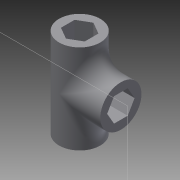
# Autodesk Inventor part: engancheBicsT
Saved by Autodesk Inventor 2015 SP1 (Build 190203100, 203)
## iProperties
Created: 2015-06-15
Part Number: engancheBicsT
Material: Genérico
Document SubType Name: Modeling
Designer: Javier
Density: 1 g/cm^3
Appearance: Valor por defecto
Author: Javier
Autodesk Inventor part; units mm, degrees
ref_plane "YZ Plane" through (0, 0, 0) normal (1, 0, 0) x (0, 1, 0)
ref_plane "XZ Plane" through (0, 0, 0) normal (0, 1, 0) x (-1, 0, 0)
ref_plane "XY Plane" through (0, 0, 0) normal (0, 0, 1) x (1, 0, 0)
sketch "Boceto1" plane through (0, 0, 0) normal (0, 0, 1) x (1, 0, 0)
  circle A0 centre (0, 0) radius 6
  line L0 (0, -4) -> (-3.4641, -2)
  line L1 (-3.4641, -2) -> (-3.4641, 2)
  line L2 (-3.4641, 2) -> (0, 4)
  line L3 (0, 4) -> (3.4641, 2)
  line L4 (3.4641, 2) -> (3.4641, -2)
  line L5 (3.4641, -2) -> (0, -4)
  dimension "d0" = 12
  dimension "d1" = 4
  constraints: 12 end point, 2 coincident, 1 centre point, 13 other
  measures "d0" diameter of A0
  measures "d1" distance of L3.end L4.end
extrude "Extrusión1" add sketch "Boceto1" along normal blind 7
sketch "Boceto2" plane through (0, 0, 7) normal (0, 0, 1) x (1, 0, 0)
  point P0 (0, 0)
sketch "Boceto3" plane through (0, 0, 7) normal (0, 0, 1) x (1, 0, 0)
  line L0 (-3.4641, -2) -> (-3.4641, 2) projected
  line L1 (-3.4641, 2) -> (0, 4) projected
  line L2 (0, 4) -> (3.4641, 2) projected
  line L3 (3.4641, 2) -> (3.4641, -2) projected
  line L4 (3.4641, -2) -> (0, -4) projected
  line L5 (0, -4) -> (-3.4641, -2) projected
  circle A0 centre (0, 0) radius 6 projected
extrude "Extrusión2" add sketch "Boceto3" along normal blind 12
ref_plane "Plano de trabajo1" through (0, -4, 19) normal (-1, 0, 0) x (0, 1, 0)
sketch "Boceto4" plane through (0, -4, 19) normal (-1, 0, 0) x (0, 1, 0)
  line L0 (8, 19) -> (8, 0) projected
  line L1 (0, 19) -> (0, 0) projected
  line L2 (6, 19) -> (2, 19) projected
  line L3 (6, 19) -> (6, 0) projected
  line L4 (2, 0) -> (6, 0) projected
  line L5 (2, 19) -> (2, 0) projected
  line L6 (2, 0) -> (6, 0)
  line L7 (4, 0) -> (4, 6)
  circle A0 centre (4, 6) radius 6
  line L8 (8, 6) -> (6, 2.5359)
  line L9 (6, 2.5359) -> (2, 2.5359)
  line L10 (2, 2.5359) -> (0, 6)
  line L11 (0, 6) -> (2, 9.4641)
  line L12 (2, 9.4641) -> (6, 9.4641)
  line L13 (6, 9.4641) -> (8, 6)
  circle A1 centre (4, 6) radius 4
  point P0 (4, 19)
  dimension "d6" = 6
  dimension "d7" = 12
  constraints: 16 end point, 3 coincident, 1 centre point, 1 midpoint, 1 perpendicular, 1 point on line, 1 vertical, 16 other
  measures "d6" distance of L7.start L7.end
  measures "d7" diameter of A0
extrude "Extrusión3" add sketch "Boceto4" against normal blind 12 contours A0 L0 | L0 A1 L3 A0 | L0 A0 L3 A1 | L3 A1 L5 A0 | L3 A0 L7 A1 | L5 A1 L1 A0 | L7 A0 L5 A1 | L1 A0 | L5 A0 L1 A1
sketch "Boceto7" plane through (0, 0, 19) normal (0, 0, 1) x (1, 0, 0)
  circle A0 centre (0, 0) radius 4
  point P0 (0, 4)
  constraints: 1 coincident, 1 vertical alignment, 2 other
extrude "Extrusión6" cut sketch "Boceto7" against normal blind 12
sketch "Boceto8" plane through (0, -4, 19) normal (-1, 0, 0) x (0, 1, 0)
  point P0 (4, 19)
sketch "Boceto9" plane through (12, 0, 13) normal (1, 0, 0) x (0, 0, -1)
  spline S0 degree 5 poles (-4, 0) (-3.9998, 1.0287) (-3.67, 2.0581) (-3.006, 2.9436) (-1.3134, 4.0903) (0.7107, 4.1022) (1.6429, 3.8257) (3.423, 2.6512) (4.2083, 0.6219) (4.2089, -0.6181) (3.4253, -2.6483) (1.6458, -3.8245) (0.7135, -4.1019) (-1.3114, -4.0911) (-3.0051, -2.9448) (-3.6697, -2.0589) (-3.9998, -1.0291) (-4, 0) knots 0 0 0 0 0 0 0.204671 0.204671 0.204671 0.387185 0.387185 0.387185 0.61267 0.61267 0.61267 0.795245 0.795245 0.795245 1 1 1 1 1 1 projected
  point P0 (13, 0)
  constraints: 1 other
extrude "Extrusión7" cut sketch "Boceto9" against normal blind 12
sketch "Boceto10" plane through (0, 0, 19) normal (0, 0, 1) x (1, 0, 0)
  circle A0 centre (0, 0) radius 6 projected
  line L0 (0, 4) -> (-3.4641, 2) projected
  line L1 (-3.4641, 2) -> (-3.4641, -2) projected
  line L2 (-3.4641, -2) -> (0, -4) projected
  line L3 (0, -4) -> (3.4641, -2) projected
  line L4 (3.4641, -2) -> (3.4641, 2) projected
  line L5 (3.4641, 2) -> (0, 4) projected
  point P0 (6, 0)
  constraints: 1 horizontal alignment
extrude "Extrusión8" add sketch "Boceto10" along normal blind 7
sketch "Boceto11" plane through (12, 0, 13) normal (1, 0, 0) x (0, 0, -1)
  circle A0 centre (0, 0) radius 4 projected
  circle A1 centre (0, 0) radius 6 projected
  line L0 (0, 4) -> (3.4641, 2)
  line L1 (3.4641, 2) -> (3.4641, -2)
  line L2 (3.4641, -2) -> (0, -4)
  line L3 (0, -4) -> (-3.4641, -2)
  line L4 (-3.4641, -2) -> (-3.4641, 2)
  line L5 (-3.4641, 2) -> (0, 4)
  point P0 (13, 0)
  constraints: 12 end point, 1 coincident, 1 vertical alignment, 14 other
extrude "Extrusión9" add sketch "Boceto11" against normal blind 7 contours A0 L1 | L0 A0 | A0 L2 | L5 A0 | A0 L3 | L4 A0
fillet "Empalme1" radius 6 4 edges at (4.2426, -4.2426, 17.2426) (4.2426, 4.2426, 17.2426) (4.2426, -4.2426, 8.7574) (4.2426, 4.2426, 8.7574)
